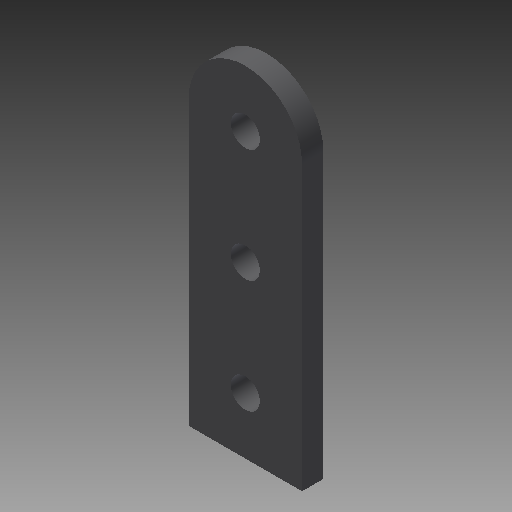
# Autodesk Inventor part: 4196
Saved by Autodesk Inventor 2017 SP1 (Build 210196100, 196)
## iProperties
Category: PARTsolutions
Company: 8020
Created: 2016-04-17
Part Number: 4196
Catalog Web Link: www.cadenas.de
Description: 4196, 4396-Joining Plates - 3 Inch Pivot Arm / 4.5 Inch Pivot Arm
Vendor: 8020
Document SubType Name: Modeling
Designer: psAdmin
Manufacturer: 8020
Mass: 8.43229 g
Surface Area: 47.4375 cm^2
Volume: 8.43229 cm^3
Density: 1 g/cm^3
Material: Generic
Appearance: PSOLRGB-192-192-192
PSOL_IDENT_0: {$CADENAS_DATA\23d-libs\8020\inch\joining_plates\4196.prj},145 {VTYP=3D},{NB=4196},{LINA=4196},{NN=4
PSOL_IDENT_1: 196, 4396},{DATE=22.08.2012},{GEOMDATE=16.01.2012 00:00:00},{VERSION=},{LINEID=10},{LINESUBID=-1},{W
PSOL_IDENT_2: BVAR=}  {NB=4196},{LINA=4196},{KT=DUMMY},{PN=4196},{A=1.000},{B=3.000},{C=0.500},{D=1.000},{E=0.500}
PSOL_IDENT_3: ,{T=0.188},{DIA=0.257},{W=.050}
NN: 4196, 4396
NT: Joining Plates - 3 Inch Pivot Arm / 4.5 Inch Pivot Arm
NB: 4196
NBSYN: $PN.
LINA: 4196
PN: 4196
A: 1.000
B: 3.000
C: 0.500
D: 1.000
E: 0.500
T: 0.188
DIA: 0.257
W: .050
SUPPLIER: 8020
ARTICLENO: 4196
BOMINFO: 4196
CREATOR: CADENAS GmbH
Title: 4196
Author: Cadenas PARTsolutions
Comments: Joining Plates - 3 Inch Pivot Arm / 4.5 Inch Pivot Arm
Autodesk Inventor part; units mm, degrees
sketch "Sketch_1" plane through (0, 0, 0) normal (0, 0, 1) x (1, 0, 0)
  line L0 (-12.7, 63.5) -> (-12.7, 0)
  line L1 (-12.7, 0) -> (12.7, 0)
  line L2 (12.7, 0) -> (12.7, 63.5)
  arc A0 (12.7, 63.5) -> (-12.7, 63.5) centre (0, 63.5) ccw
  circle A1 centre (0, 12.7) radius 3.2639
  circle A2 centre (0, 38.1) radius 3.2639
  circle A3 centre (0, 63.5) radius 3.2639
  constraints: 6 end point, 4 centre point, 2 point on circle
extrude "Extrusion1" add sketch "Sketch_1" along normal blind 4.7752
ref_plane "pivot_arm_XY" through (0, 63.5, 0) normal (0, 0, 1) x (1, 0, 0)
ref_plane "pivot_arm_YZ" through (0, 63.5, 0) normal (1, 0, 0) x (0, 1, 0)
ref_plane "pivot_arm_ZX" through (0, 63.5, 0) normal (0, 1, 0) x (0, 0, 1)
ref_plane "to_bolt_XY" through (0, 63.5, 4.7752) normal (0, 0, 1) x (1, 0, 0)
ref_plane "to_bolt_YZ" through (0, 63.5, 4.7752) normal (1, 0, 0) x (0, 1, 0)
ref_plane "to_bolt_ZX" through (0, 63.5, 4.7752) normal (0, 1, 0) x (0, 0, 1)
body "Solid1"
